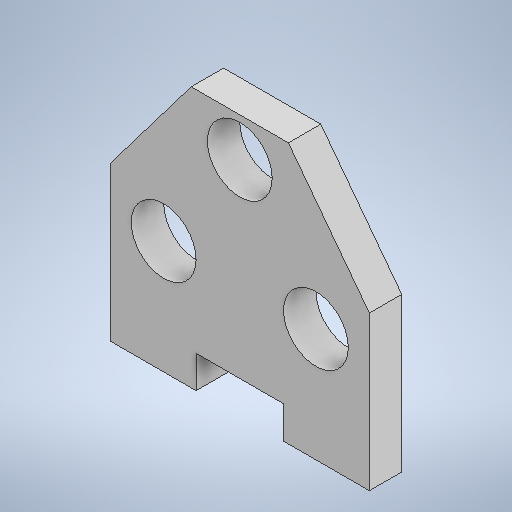
# Autodesk Inventor part: Project_support_stand
Saved by Autodesk Inventor 2025 (Build 290162000, 162)
## iProperties
Created: 2025-08-31
Part Number: Project_support_stand
Material: Generic
Document SubType Name: Modeling
Designer: Kiran
Density: 1 g/cm^3
Appearance: Default
Author: Kiran
Autodesk Inventor part; units mm, degrees
ref_plane "YZ Plane" through (0, 0, 0) normal (1, 0, 0) x (0, 1, 0)
ref_plane "XZ Plane" through (0, 0, 0) normal (0, 1, 0) x (-1, 0, 0)
ref_plane "XY Plane" through (0, 0, 0) normal (0, 0, 1) x (1, 0, 0)
sketch "Sketch1" plane through (0, 0, 0) normal (0, 0, 1) x (1, 0, 0)
  line L0 (-80, 0) -> (80, 0)
  line L1 (80, 0) -> (80, 50)
  line L2 (-80, 50) -> (-80, 0)
  line L3 (0, 116) -> (30, 116)
  line L4 (30, 116) -> (-30, 116)
  line L5 (-30, 116) -> (-80, 50)
  line L6 (30, 116) -> (80, 50)
  circle A0 centre (0, 92) radius 8
  circle A1 centre (0, 92) radius 12
  line L7 (80, 0) -> (80, -15)
  line L8 (80, -15) -> (55, -15)
  line L9 (55, -15) -> (55, 0)
  line L10 (-80, 0) -> (-80, -15)
  line L11 (-80, -15) -> (-55, -15)
  line L12 (-55, -15) -> (-55, 0)
  circle A2 centre (47, 25) radius 20
  circle A3 centre (-47, 25) radius 20
  circle A4 centre (0, 92) radius 20
  point P0 (0, 0)
  dimension "d0" = 160
  dimension "d1" = 50
  dimension "d3" = 60
  dimension "d4" = 16
  dimension "d5" = 24
  dimension "d6" = 15
  dimension "d7" = 25
  dimension "d12" = 40
  dimension "d13" = 40
  dimension "d21" = 40
  constraints: 26 end point, 5 centre point, 4 perpendicular, 3 point on line, 3 vertical, 2 coincident, 2 horizontal
  measures "d0" distance of L0.start L0.end
  measures "d1" distance of L0.end L1.end
  measures "d3" distance of L3.end L4.end
  measures "d4" diameter of A0
  measures "d5" diameter of A1
  measures "d6" distance of L0.end L7.end
  measures "d7" distance of L7.end L8.end
  measures "d12" diameter of A2
  measures "d13" diameter of A3
  measures "d21" diameter of A4
extrude "Extrusion1" add sketch "Sketch1" along normal blind 20 contours L2 L5 L4 L3 L6 L1 L0 | L0 L12 L11 L10 | L0 L7 L8 L9 | A1 | A4
sketch "Sketch5" plane through (0, 0, 0) normal (0, 0, -1) x (-1, 0, 0)
  circle A0 centre (0, 92) radius 8 projected
  circle A1 centre (0, 92) radius 20
  point P0 (0, 0)
  dimension "d22" = 40
  constraints: 1 centre point, 1 coincident
  measures "d22" diameter of A1
extrude "Extrusion4" cut sketch "Sketch5" against normal blind 20
sketch "Sketch6" plane through (-55, 0, 0) normal (0, -1, 0) x (1, 0, 0)
  point P0 (55, 0)
sketch "Sketch7" plane through (-55, 0, 0) normal (0, -1, 0) x (1, 0, 0)
  line L0 (-25, 0) -> (-25, 20) projected
  line L1 (-12, 0) -> (28, 0) projected
  line L2 (-25, 20) -> (28, 20)
  line L3 (28, 20) -> (28, 0)
  line L4 (28, 0) -> (-25, 0)
  line L5 (-25, 0) -> (-25, 20)
  line L6 (135, 0) -> (135, 20) projected
  line L7 (135, 20) -> (82, 20)
  line L8 (82, 20) -> (82, 0)
  line L9 (82, 0) -> (135, 0)
  line L10 (135, 0) -> (135, 20)
  point P0 (55, 0)
  dimension "d25" = 53
  constraints: 16 end point, 4 parallel, 2 horizontal, 2 perpendicular, 1 point on line
  measures "d25" distance of L9.end L8.end
extrude "Extrusion5" add sketch "Sketch7" along normal blind 45
sketch "Sketch8" plane through (-27, 0, 0) normal (0, -1, 0) x (1, 0, 0)
  line L0 (-40, 20) -> (0, 20) projected
  line L1 (57, 0) -> (-3, 0) projected
  line L2 (0, 20) -> (54, 20)
  line L3 (54, 20) -> (54, 0)
  line L4 (54, 0) -> (0, 0)
  line L5 (0, 0) -> (0, 20)
  point P0 (27, 0)
  constraints: 8 end point, 2 parallel, 1 horizontal, 1 perpendicular, 1 point on line
extrude "Extrusion6" add sketch "Sketch8" along normal blind 25
body "Solid1"
